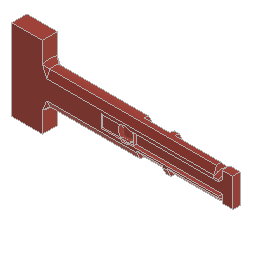
Protec2 (Autodesk Fusion 360 design; units mm, degrees)
Autodesk Fusion 360 part; units mm, degrees
sketch "profile" plane through (0, 0, 0) normal (1, 0, 0) x (0, 1, 0)
  line L0 (0, 0) -> (3.3, 0) construction
  line L1 (3.3, 0) -> (3.3, 3.3) construction
  line L2 (3.3, 3.3) -> (4.05, 3.3) construction
  line L3 (3.3, 3.3) -> (2.55, 3.3) construction
  line L4 (4.05, 3.3) -> (4.05, 4.5)
  line L5 (2.55, 3.3) -> (2.55, 2.1)
  line L6 (4.05, 3.3) -> (4.05, 2.1)
  line L7 (2.55, 3.3) -> (2.55, 4.5)
  line L8 (4.05, 4.5) -> (4.775, 4.5)
  line L9 (2.55, 2.1) -> (1.825, 2.1)
  line L10 (4.05, 2.1) -> (4.775, 2.1)
  line L11 (2.55, 4.5) -> (1.825, 4.5)
  line L12 (4.775, 4.5) -> (4.775, 5.165)
  line L13 (1.825, 2.1) -> (1.825, 1.435)
  line L14 (1.825, 4.5) -> (1.825, 5.165)
  line L15 (4.775, 2.1) -> (4.775, 1.435)
  line L16 (4.775, 5.165) -> (4.1589, 6.4863)
  line L17 (4.775, 5.165) -> (3.3, 5.165) construction
  line L18 (1.825, 1.435) -> (2.4411, 0.1137)
  line L19 (1.825, 5.165) -> (2.4411, 6.4863)
  line L20 (1.825, 5.165) -> (3.3, 5.165) construction
  line L21 (4.775, 1.435) -> (4.1589, 0.1137)
  arc A0 (4.1589, 6.4863) -> (2.4411, 6.4863) centre (3.3, 3.3) ccw
  arc A1 (2.4411, 0.1137) -> (4.1589, 0.1137) centre (3.3, 3.3) ccw
  dimension "d64" = 3.3
  dimension "d65" = 3.3
  dimension "d66" = 0.75
  dimension "d67" = 0.75
  dimension "d68" = 1.2
  dimension "d69" = 1.2
  dimension "d70" = 1.2
  dimension "d71" = 1.2
  dimension "d72" = 0.725
  dimension "d73" = 0.725
  dimension "d74" = 0.725
  dimension "d75" = 0.725
  dimension "d76" = 65
  dimension "d77" = 65
  dimension "d78" = 4.25
  dimension "d79" = 4.25
  dimension "d80" = 3.3
  constraint coincident L0.start origin
  constraint horizontal L0
  constraint perpendicular L0 L1
  constraint perpendicular L1 L2
  constraint perpendicular L1 L3
  constraint perpendicular L2 L4
  constraint perpendicular L3 L5
  constraint perpendicular L2 L6
  constraint perpendicular L3 L7
  constraint perpendicular L4 L8
  constraint perpendicular L5 L9
  constraint perpendicular L6 L10
  constraint perpendicular L7 L11
  constraint perpendicular L8 L12
  constraint perpendicular L9 L13
  constraint equal L12 L13
  constraint perpendicular L11 L14
  constraint perpendicular L10 L15
  constraint equal L14 L15
  constraint horizontal L17
  constraint equal L16 L18
  constraint parallel L16 L18
  constraint vertical L1.end L17.end
  constraint horizontal L20
  constraint equal L19 L21
  constraint parallel L19 L21
  constraint coincident L1.end L2.start
  constraint coincident L16.end A0.start
  measures "d64" distance of L0.start L0.end
  measures "d65" distance of L0.end L1.end
  measures "d66" distance of L1.end L2.end
  measures "d67" distance of L1.end L3.end
  measures "d68" distance of L2.end L4.end
  measures "d69" distance of L3.end L5.end
  measures "d70" distance of L2.end L6.end
  measures "d71" distance of L3.end L7.end
  measures "d72" distance of L4.end L8.end
  measures "d73" distance of L5.end L9.end
  measures "d74" distance of L6.end L10.end
  measures "d75" distance of L7.end L11.end
  measures "d76" angle of L16 L17
  measures "d77" angle of L19 L20
  measures "d78" distance of L16 L18
  measures "d79" distance of L19 L21
  measures "d80" radius of A0
extrude "Extrude1" add sketch "profile" against normal blind 42.57 makes body 1
ref_plane "WorkPlane1" through (-21.285, 3.3, 3.3) normal (0, -1, 0) x (0, 0, 1)
sketch "bearing hole" plane through (0, 3.3, 0) normal (0, -1, 0) x (-1, 0, 0)
  line L0 (0, 0) -> (0, -3.3) construction
  line L1 (0, -3.3) -> (20.5, -3.3) construction
  circle A0 centre (20.5, -3.3) radius 1.5
  dimension "d83" = 3.3
  dimension "d84" = 20.5
  dimension "d85" = 3
  constraint coincident L0.start origin
  constraint vertical L0
  constraint perpendicular L0 L1
  constraint coincident L1.end A0.centre
  measures "d83" distance of L0.start L0.end
  measures "d84" distance of L0.end L1.end
  measures "d85" diameter of A0
ref_plane "WorkPlane2" through (-42.57, 0, 0) normal (1, 0, 0) x (0, 1, 0)
sketch "bow" plane through (-42.57, 0, 0) normal (1, 0, 0) x (0, 1, 0)
  circle A0 centre (3.3, 3.3) radius 3.3 construction
  line L0 (4.775, 5.165) -> (4.775, 6.252)
  line L1 (4.775, 1.435) -> (4.775, 0.348)
  line L2 (1.825, 1.435) -> (1.825, 0.348)
  line L3 (1.825, 5.165) -> (1.825, 6.252)
  line L4 (4.775, 5.165) -> (4.775, 1.435)
  line L5 (1.825, 5.165) -> (1.825, 1.435)
  line L6 (4.775, 6.252) -> (4.775, 11.252)
  line L7 (1.825, 0.348) -> (1.825, -4.652)
  line L8 (4.775, 11.252) -> (1.825, 11.252)
  line L9 (1.825, 11.252) -> (1.825, 6.252)
  line L10 (1.825, -4.652) -> (4.775, -4.652)
  line L11 (4.775, -4.652) -> (4.775, 0.348)
  line L12 (2.55, 2.1) -> (2.55, 4.5) construction
  line L13 (2.55, 4.5) -> (1.825, 4.5) construction
  line L14 (1.825, 4.5) -> (1.825, 5.165) construction
  line L15 (1.825, 5.165) -> (2.4411, 6.4863) construction
  arc A1 (4.1589, 6.4863) -> (2.4411, 6.4863) centre (3.3, 3.3) ccw construction
  line L16 (4.1589, 6.4863) -> (4.775, 5.165) construction
  line L17 (4.775, 5.165) -> (4.775, 4.5) construction
  line L18 (4.775, 4.5) -> (4.05, 4.5) construction
  line L19 (4.05, 4.5) -> (4.05, 2.1) construction
  line L20 (4.05, 2.1) -> (4.775, 2.1) construction
  line L21 (4.775, 2.1) -> (4.775, 1.435) construction
  line L22 (4.775, 1.435) -> (4.1589, 0.1137) construction
  arc A2 (2.4411, 0.1137) -> (4.1589, 0.1137) centre (3.3, 3.3) ccw construction
  line L23 (2.4411, 0.1137) -> (1.825, 1.435) construction
  line L24 (1.825, 1.435) -> (1.825, 2.1) construction
  line L25 (1.825, 2.1) -> (2.55, 2.1) construction
  dimension "d86" = 5
  dimension "d87" = 5
  constraint coincident A0 L0.end
  constraint coincident A0 L1.end
  constraint coincident A0 L2.end
  constraint coincident A0 L3.end
  constraint parallel L0 L6
  constraint parallel L2 L7
  constraint perpendicular L3 L8
  constraint perpendicular L8 L9
  constraint perpendicular L1 L10
  constraint perpendicular L10 L11
  constraint coincident L0.start L4.start
  constraint coincident A0 A1.start
  constraint coincident A0 L15.end
  constraint coincident A0 A2.start
  constraint vertical L9
  constraint vertical L6
  constraint vertical L11
  constraint vertical L7
  constraint vertical L4
  constraint vertical L5
  constraint coincident L2.start L5.end
  constraint coincident L3.start L5.start
  constraint coincident L1.start L4.end
  measures "d86" distance of L0.end L6.end
  measures "d87" distance of L2.end L7.end
sketch "bearing hole and shaft strength" plane through (-42.57, 0, 0) normal (1, 0, 0) x (0, 1, 0)
  line L0 (2.55, 2.1) -> (2.55, 4.5)
  line L1 (4.05, 4.5) -> (4.05, 2.1)
  line L2 (2.55, 4.5) -> (1.825, 4.5)
  line L3 (1.825, 2.1) -> (2.55, 2.1)
  line L4 (4.05, 2.1) -> (4.775, 2.1)
  line L5 (4.775, 4.5) -> (4.05, 4.5)
  line L6 (2.125, 4.5) -> (2.125, 2.1)
  line L7 (4.475, 4.5) -> (4.475, 2.1)
  line L8 (1.825, 4.5) -> (1.825, 2.1)
  line L9 (4.775, 2.1) -> (4.775, 4.5)
  dimension "d89" = 0.425
  dimension "d90" = 0.425
  constraint coincident L2 L6.start
  constraint coincident L3 L6.end
  constraint perpendicular L3 L6
  constraint coincident L5 L7.start
  constraint coincident L4 L7.end
  constraint perpendicular L4 L7
  constraint coincident L2.end L8.start
  constraint coincident L3.start L8.end
  constraint coincident L4.end L9.start
  constraint coincident L5.start L9.end
  measures "d89" distance of L0 L6
  measures "d90" distance of L1 L7
extrude "Extrude2" add sketch "bow" along normal blind 6 bodies 1
extrude "Extrude3" add sketch "bearing hole and shaft strength" along normal blind 23.625 contours L0 L2 L3 L6 | L1 L4 L5 L7 bodies 1
extrude "Extrude4" add sketch "bearing hole and shaft strength" along normal blind 17.5 contours L2 L3 L6 L8 | L4 L5 L7 L9 bodies 1
chamfer "Chamfer1" distance 0.85 angle 45 6 edges at (-36.57, 2.1331, 5.8256) (-36.57, 3.3, 6.6) (-36.57, 2.1331, 0.7744) (-36.57, 4.4669, 5.8256) (-36.57, 4.4669, 0.7744) (-36.57, 3.3, 0) on bodies 1
extrude "Extrude5" cut sketch "bearing hole" along normal through all and the other way through all bodies 1
sketch "bearing" plane through (0, 3.3, 0) normal (0, -1, 0) x (-1, 0, 0)
  circle A0 centre (20.5, -3.3) radius 1.25
  point P0 (20.5, -3.3)
  dimension "d99" = 2.5
  constraint coincident P0 A0.centre
  measures "d99" diameter of A0
ref_plane "WorkPlane3" through (-20.5, 4.775, 3.3) normal (-1, 0, 0) x (0, -1, 0)
sketch "bearing post" plane through (-20.5, 0, 0) normal (-1, 0, 0) x (0, -1, 0)
  circle A0 centre (-3.3, 3.3) radius 0.3
  point P0 (-3.3, 3.3)
  dimension "d105" = 0.6
  constraint coincident P0 A0.centre
  measures "d105" diameter of A0
extrude "Extrude6" add sketch "bearing" along normal mid plane 2.5 separate body makes body 2
fillet "Fillet1" radius 1.25 2 edges at (-19.3346, 2.05, 3.752) (-19.3346, 4.55, 2.848) on bodies 2
extrude "Extrude7" add sketch "bearing post" along normal up to surface end surface at (-21.2817, 3.6917, 4.5802) on bodies 1 bodies 1 2
sketch "bearing retention" plane through (0, 2.125, 0) normal (0, -1, 0) x (1, 0, 0)
  arc A0 (-21.4, 4.5) -> (-21.4, 2.1) centre (-20.5, 3.3) ccw
  line L0 (-21.4, 4.5) -> (-25.07, 4.5)
  line L1 (-25.07, 4.5) -> (-25.07, 2.1)
  line L2 (-25.07, 2.1) -> (-21.4, 2.1)
  arc A1 (-21.4, 2.1) -> (-19.6, 2.1) centre (-20.5, 3.3) ccw
  arc A2 (-19.6, 4.5) -> (-21.4, 4.5) centre (-20.5, 3.3) ccw
  line L3 (-21.3292, 2.05) -> (-19.6708, 2.05) construction
  line L4 (-21.3292, 2.05) -> (-21.3292, 2.225)
  line L5 (-21.3292, 2.225) -> (-19.6708, 2.225)
  line L6 (-19.6708, 2.225) -> (-19.6708, 2.05)
  line L7 (-21.3292, 4.55) -> (-19.6708, 4.55) construction
  line L8 (-21.3292, 4.55) -> (-21.3292, 4.375)
  line L9 (-21.3292, 4.375) -> (-19.6708, 4.375)
  line L10 (-19.6708, 4.375) -> (-19.6708, 4.55)
  point P0 (-20.5, 1.8)
  point P1 (-20.5, 4.8)
  dimension "d108" = 0.25
  dimension "d109" = 0.175
  dimension "d110" = 0.175
  constraint midpoint A2 P1
  constraint coincident A1 L3.start
  constraint coincident A1 L3.end
  constraint horizontal L3
  constraint perpendicular L3 L4
  constraint perpendicular L4 L5
  constraint perpendicular L3 L6
  constraint coincident A2 L7.start
  constraint coincident A2 L7.end
  constraint horizontal L7
  constraint equal L3 L7
  constraint perpendicular L7 L8
  constraint perpendicular L8 L9
  constraint perpendicular L7 L10
  constraint midpoint A1 P0
  measures "d108" distance of P0 L3
  measures "d109" distance of L3.start L4.end
  measures "d110" distance of L7.start L8.end
extrude "Extrude8" add sketch "bearing retention" against normal blind 0.35 contours A1 L4 L5 L6 | A2 L8 L9 L10 bodies 1
fillet "Fillet2" radius 0.175 2 faces at (-20.7764, 2.2417, 2.225) (-20.7764, 2.2417, 4.375) on bodies 1
mirror "Mirror1" about plane through (-21.285, 3.3, 3.3) normal (0, -1, 0) of "Extrude8", "Fillet2"
sketch "tip" plane through (0, 0, 0) normal (1, 0, 0) x (0, 1, 0)
  line L0 (0, 0) -> (3.3, 0) construction
  line L1 (3.3, 0) -> (3.3, 3.3) construction
  line L2 (3.3, 3.3) -> (4.05, 3.3) construction
  line L3 (3.3, 3.3) -> (2.55, 3.3) construction
  line L4 (4.05, 3.3) -> (4.05, 6.1013)
  line L5 (2.55, 3.3) -> (2.55, 0.4987)
  line L6 (4.05, 3.3) -> (4.05, 0.4987)
  line L7 (2.55, 3.3) -> (2.55, 6.1013)
  arc A0 (4.05, 6.1013) -> (2.55, 6.1013) centre (3.3, 3.3) ccw
  arc A1 (2.55, 0.4987) -> (4.05, 0.4987) centre (3.3, 3.3) ccw
  circle A2 centre (3.3, 3.3) radius 3.3
  dimension "d117" = 3.3
  dimension "d118" = 3.3
  dimension "d119" = 0.75
  dimension "d120" = 0.75
  dimension "d121" = 2.9
  dimension "d122" = 6.6
  constraint coincident L0.start origin
  constraint horizontal L0
  constraint perpendicular L0 L1
  constraint perpendicular L1 L2
  constraint perpendicular L1 L3
  constraint perpendicular L2 L4
  constraint perpendicular L3 L5
  constraint perpendicular L2 L6
  constraint perpendicular L3 L7
  constraint equal L5 L7
  constraint equal L6 L7
  constraint equal L4 L6
  constraint coincident L1.end L2.start
  constraint concentric A0 A2
  measures "d117" distance of L0.start L0.end
  measures "d118" distance of L0.end L1.end
  measures "d119" distance of L1.end L2.end
  measures "d120" distance of L1.end L3.end
  measures "d121" radius of A0
  measures "d122" diameter of A2
sketch "profiled 0 cut" plane through (0, 0, 0) normal (1, 0, 0) x (0, 1, 0)
  line L0 (2.55, 4.5) -> (1.825, 4.5)
  line L1 (2.55, 3.3) -> (2.55, 4.5)
  line L2 (2.55, 3.3) -> (2.55, 2.1)
  line L3 (2.55, 2.1) -> (1.825, 2.1)
  line L4 (4.05, 3.3) -> (4.05, 4.5)
  line L5 (4.05, 4.5) -> (4.775, 4.5)
  line L6 (4.05, 3.3) -> (4.05, 2.1)
  line L7 (4.05, 2.1) -> (4.775, 2.1)
  line L8 (4.775, 4.5) -> (4.775, 4.8293)
  line L9 (1.825, 2.1) -> (1.825, 1.7707)
  line L10 (4.775, 2.1) -> (4.775, 1.7707)
  line L11 (1.825, 4.5) -> (1.825, 4.8293)
  line L12 (4.775, 4.8293) -> (4.7747, 4.83)
  line L13 (4.775, 4.8293) -> (3.3, 4.8293) construction
  line L14 (1.825, 1.7707) -> (1.8253, 1.77)
  line L15 (1.825, 4.8293) -> (1.8253, 4.83)
  line L16 (1.825, 4.8293) -> (3.3, 4.8293) construction
  line L17 (4.775, 1.7707) -> (4.7747, 1.77)
  arc A0 (4.7747, 4.83) -> (1.8253, 4.83) centre (3.3, 3.3) ccw
  arc A1 (1.8253, 1.77) -> (4.7747, 1.77) centre (3.3, 3.3) ccw
  circle A2 centre (3.3, 3.3) radius 4.125
  point P0 (3.3, 3.3)
  dimension "d153" = 65
  dimension "d154" = 65
  dimension "d155" = 3.9663
  dimension "d156" = 3.9663
  dimension "d157" = 2.125
  dimension "d158" = 8.25
  constraint coincident L5.end L8.start
  constraint perpendicular L5 L8
  constraint coincident L3.end L9.start
  constraint perpendicular L3 L9
  constraint equal L8 L9
  constraint coincident L7.end L10.start
  constraint perpendicular L7 L10
  constraint coincident L0.end L11.start
  constraint perpendicular L0 L11
  constraint equal L10 L11
  constraint horizontal L13
  constraint vertical P0 L13.end
  constraint equal L12 L14
  constraint parallel L12 L14
  constraint horizontal L16
  constraint equal L15 L17
  constraint parallel L15 L17
  constraint coincident P0 A0.centre
  constraint coincident L12.end A0.start
  measures "d153" angle of L12 L13
  measures "d154" angle of L15 L16
  measures "d155" distance of L12 L14
  measures "d156" distance of L15 L17
  measures "d157" radius of A0
  measures "d158" diameter of A2
sketch "Sketch9" plane through (0, 0, 0) normal (1, 0, 0) x (0, 1, 0)
  line L0 (4.05, 4.5) -> (4.775, 4.5)
  line L1 (4.05, 3.3) -> (4.05, 4.5)
  line L2 (4.05, 3.3) -> (4.05, 2.1)
  line L3 (4.05, 2.1) -> (4.775, 2.1)
  line L4 (2.55, 2.1) -> (1.825, 2.1)
  line L5 (2.55, 3.3) -> (2.55, 2.1)
  line L6 (2.55, 3.3) -> (2.55, 4.5)
  line L7 (2.55, 4.5) -> (1.825, 4.5)
  line L8 (4.775, 4.5) -> (4.775, 4.8481)
  line L9 (1.825, 2.1) -> (1.825, 1.7519)
  line L10 (4.775, 4.8481) -> (3.305, 6.6)
  line L11 (4.775, 4.8481) -> (3.3, 4.8481) construction
  line L12 (1.825, 1.7519) -> (3.295, 0)
  line L13 (1.825, 4.5) -> (1.825, 5.165)
  line L14 (4.775, 2.1) -> (4.775, 1.435)
  line L15 (1.825, 5.165) -> (2.4411, 6.4863)
  line L16 (1.825, 5.165) -> (3.3, 5.165) construction
  line L17 (4.775, 1.435) -> (4.1589, 0.1137)
  arc A0 (3.305, 6.6) -> (2.4411, 6.4863) centre (3.3, 3.3) ccw
  arc A1 (3.295, 0) -> (4.1589, 0.1137) centre (3.3, 3.3) ccw
  circle A2 centre (3.3, 3.3) radius 4.125
  point P0 (3.3, 3.3)
  dimension "d123" = 50
  dimension "d124" = 65
  dimension "d125" = 3.3
  dimension "d126" = 4.25
  dimension "d127" = 4.25
  dimension "d128" = 8.25
  constraint coincident L0.end L8.start
  constraint perpendicular L0 L8
  constraint coincident L4.end L9.start
  constraint perpendicular L4 L9
  constraint equal L8 L9
  constraint horizontal L11
  constraint vertical P0 L11.end
  constraint parallel L10 L12
  constraint coincident L7.end L13.start
  constraint perpendicular L7 L13
  constraint coincident L3.end L14.start
  constraint perpendicular L3 L14
  constraint equal L13 L14
  constraint horizontal L16
  constraint parallel L15 L17
  constraint equal L15 L17
  constraint equal L10 L12
  constraint coincident P0 A0.centre
  constraint coincident L10.end A0.start
  constraint equal A0 A1
  constraint vertical L16.end P0
  constraint concentric A0 A2
  measures "d123" angle of L10 L11
  measures "d124" angle of L15 L16
  measures "d125" radius of A0
  measures "d126" distance of L10 L12
  measures "d127" distance of L15 L17
  measures "d128" diameter of A2
sketch "Sketch10" plane through (0, 0, 0) normal (1, 0, 0) x (0, 1, 0)
  line L0 (2.55, 4.5) -> (1.825, 4.5)
  line L1 (2.55, 3.3) -> (2.55, 4.5)
  line L2 (4.05, 4.5) -> (4.775, 4.5)
  line L3 (4.05, 3.3) -> (4.05, 4.5)
  line L4 (4.05, 2.1) -> (4.775, 2.1)
  line L5 (4.05, 3.3) -> (4.05, 2.1)
  line L6 (2.55, 3.3) -> (2.55, 2.1)
  line L7 (2.55, 2.1) -> (1.825, 2.1)
  line L8 (4.775, 4.5) -> (4.775, 4.8481)
  line L9 (1.825, 2.1) -> (1.825, 1.7519)
  line L10 (1.825, 4.5) -> (1.825, 5.165)
  line L11 (4.775, 2.1) -> (4.775, 1.435)
  line L12 (4.775, 4.8481) -> (3.305, 6.6)
  line L13 (4.775, 4.8481) -> (3.3, 4.8481) construction
  line L14 (1.825, 1.7519) -> (3.295, 0)
  line L15 (1.825, 5.165) -> (2.4411, 6.4863)
  line L16 (1.825, 5.165) -> (3.3, 5.165) construction
  line L17 (4.775, 1.435) -> (4.1589, 0.1137)
  arc A0 (3.305, 6.6) -> (2.4411, 6.4863) centre (3.3, 3.3) ccw
  arc A1 (3.295, 0) -> (4.1589, 0.1137) centre (3.3, 3.3) ccw
  circle A2 centre (3.3, 3.3) radius 4.125
  point P0 (3.3, 3.3)
  dimension "d129" = 50
  dimension "d130" = 65
  dimension "d131" = 4.25
  dimension "d132" = 4.25
  dimension "d133" = 3.3
  dimension "d134" = 8.25
  constraint coincident L2.end L8.start
  constraint perpendicular L2 L8
  constraint coincident L7.end L9.start
  constraint perpendicular L7 L9
  constraint equal L8 L9
  constraint coincident L0.end L10.start
  constraint perpendicular L0 L10
  constraint coincident L4.end L11.start
  constraint perpendicular L4 L11
  constraint equal L10 L11
  constraint horizontal L13
  constraint equal L12 L14
  constraint parallel L12 L14
  constraint vertical P0 L13.end
  constraint horizontal L16
  constraint vertical P0 L16.end
  constraint equal L15 L17
  constraint parallel L15 L17
  constraint coincident P0 A0.centre
  constraint coincident L12.end A0.start
  constraint equal A0 A1
  constraint concentric A1 A2
  measures "d129" angle of L12 L13
  measures "d130" angle of L15 L16
  measures "d131" distance of L12 L14
  measures "d132" distance of L15 L17
  measures "d133" radius of A0
  measures "d134" diameter of A2
sketch "Sketch11" plane through (0, 0, 0) normal (1, 0, 0) x (0, 1, 0)
  line L0 (4.05, 4.5) -> (4.775, 4.5)
  line L1 (4.05, 3.3) -> (4.05, 4.5)
  line L2 (4.05, 3.3) -> (4.05, 2.1)
  line L3 (4.05, 2.1) -> (4.775, 2.1)
  line L4 (2.55, 3.3) -> (2.55, 4.5)
  line L5 (2.55, 3.3) -> (2.55, 2.1)
  line L6 (2.55, 2.1) -> (1.825, 2.1)
  line L7 (2.55, 4.5) -> (1.825, 4.5)
  line L8 (4.775, 4.5) -> (4.775, 4.8481)
  line L9 (1.825, 2.1) -> (1.825, 1.7519)
  line L10 (1.825, 4.5) -> (1.825, 5.165)
  line L11 (4.775, 2.1) -> (4.775, 1.435)
  line L12 (4.775, 4.8481) -> (3.305, 6.6)
  line L13 (4.775, 4.8481) -> (3.3, 4.8481) construction
  line L14 (1.825, 1.7519) -> (3.295, 0)
  line L15 (1.825, 5.165) -> (2.4411, 6.4863)
  line L16 (1.825, 5.165) -> (3.3, 5.165) construction
  line L17 (4.775, 1.435) -> (4.1589, 0.1137)
  arc A0 (3.305, 6.6) -> (2.4411, 6.4863) centre (3.3, 3.3) ccw
  arc A1 (3.295, 0) -> (4.1589, 0.1137) centre (3.3, 3.3) ccw
  circle A2 centre (3.3, 3.3) radius 4.125
  point P0 (3.3, 3.3)
  dimension "d135" = 50
  dimension "d136" = 65
  dimension "d137" = 4.25
  dimension "d138" = 4.25
  dimension "d139" = 3.3
  dimension "d140" = 8.25
  constraint coincident L0.end L8.start
  constraint perpendicular L0 L8
  constraint coincident L6.end L9.start
  constraint perpendicular L6 L9
  constraint equal L8 L9
  constraint coincident L7.end L10.start
  constraint perpendicular L7 L10
  constraint coincident L3.end L11.start
  constraint perpendicular L3 L11
  constraint equal L10 L11
  constraint horizontal L13
  constraint parallel L12 L14
  constraint equal L12 L14
  constraint vertical P0 L13.end
  constraint horizontal L16
  constraint vertical P0 L16.end
  constraint equal L15 L17
  constraint parallel L15 L17
  constraint coincident P0 A0.centre
  constraint coincident L12.end A0.start
  constraint equal A0 A1
  constraint concentric A1 A2
  measures "d135" angle of L12 L13
  measures "d136" angle of L15 L16
  measures "d137" distance of L12 L14
  measures "d138" distance of L15 L17
  measures "d139" radius of A0
  measures "d140" diameter of A2
sketch "Sketch12" plane through (0, 0, 0) normal (1, 0, 0) x (0, 1, 0)
  line L0 (2.55, 4.5) -> (1.825, 4.5)
  line L1 (2.55, 3.3) -> (2.55, 4.5)
  line L2 (2.55, 3.3) -> (2.55, 2.1)
  line L3 (2.55, 2.1) -> (1.825, 2.1)
  line L4 (4.05, 3.3) -> (4.05, 4.5)
  line L5 (4.05, 4.5) -> (4.775, 4.5)
  line L6 (4.05, 3.3) -> (4.05, 2.1)
  line L7 (4.05, 2.1) -> (4.775, 2.1)
  line L8 (4.775, 4.5) -> (4.775, 4.8481)
  line L9 (1.825, 2.1) -> (1.825, 1.7519)
  line L10 (1.825, 4.5) -> (1.825, 5.165)
  line L11 (4.775, 2.1) -> (4.775, 1.435)
  line L12 (4.775, 4.8481) -> (3.305, 6.6)
  line L13 (4.775, 4.8481) -> (3.3, 4.8481) construction
  line L14 (1.825, 1.7519) -> (3.295, 0)
  line L15 (1.825, 5.165) -> (2.4411, 6.4863)
  line L16 (1.825, 5.165) -> (3.3, 5.165) construction
  line L17 (4.775, 1.435) -> (4.1589, 0.1137)
  arc A0 (3.305, 6.6) -> (2.4411, 6.4863) centre (3.3, 3.3) ccw
  arc A1 (3.295, 0) -> (4.1589, 0.1137) centre (3.3, 3.3) ccw
  circle A2 centre (3.3, 3.3) radius 4.125
  point P0 (3.3, 3.3)
  dimension "d141" = 50
  dimension "d142" = 65
  dimension "d143" = 4.25
  dimension "d144" = 4.25
  dimension "d145" = 3.3
  dimension "d146" = 8.25
  constraint coincident L5.end L8.start
  constraint perpendicular L5 L8
  constraint coincident L3.end L9.start
  constraint perpendicular L3 L9
  constraint equal L8 L9
  constraint coincident L0.end L10.start
  constraint perpendicular L0 L10
  constraint coincident L7.end L11.start
  constraint perpendicular L7 L11
  constraint equal L10 L11
  constraint horizontal L13
  constraint vertical P0 L13.end
  constraint equal L12 L14
  constraint parallel L12 L14
  constraint horizontal L16
  constraint vertical P0 L16.end
  constraint parallel L15 L17
  constraint equal L15 L17
  constraint coincident P0 A0.centre
  constraint coincident L12.end A0.start
  constraint equal A0 A1
  measures "d141" angle of L12 L13
  measures "d142" angle of L15 L16
  measures "d143" distance of L12 L14
  measures "d144" distance of L15 L17
  measures "d145" radius of A0
  measures "d146" diameter of A2
sketch "Sketch13" plane through (0, 0, 0) normal (1, 0, 0) x (0, 1, 0)
  line L0 (2.55, 4.5) -> (1.825, 4.5)
  line L1 (2.55, 3.3) -> (2.55, 4.5)
  line L2 (2.55, 3.3) -> (2.55, 2.1)
  line L3 (2.55, 2.1) -> (1.825, 2.1)
  line L4 (4.05, 2.1) -> (4.775, 2.1)
  line L5 (4.05, 3.3) -> (4.05, 2.1)
  line L6 (4.05, 3.3) -> (4.05, 4.5)
  line L7 (4.05, 4.5) -> (4.775, 4.5)
  line L8 (4.775, 4.5) -> (4.775, 4.8481)
  line L9 (1.825, 2.1) -> (1.825, 1.7519)
  line L10 (1.825, 4.5) -> (1.825, 5.165)
  line L11 (4.775, 2.1) -> (4.775, 1.435)
  line L12 (4.775, 4.8481) -> (3.305, 6.6)
  line L13 (4.775, 4.8481) -> (3.3, 4.8481) construction
  line L14 (1.825, 1.7519) -> (3.295, 0)
  line L15 (1.825, 5.165) -> (2.4411, 6.4863)
  line L16 (1.825, 5.165) -> (3.3, 5.165) construction
  line L17 (4.775, 1.435) -> (4.1589, 0.1137)
  arc A0 (3.305, 6.6) -> (2.4411, 6.4863) centre (3.3, 3.3) ccw
  arc A1 (3.295, 0) -> (4.1589, 0.1137) centre (3.3, 3.3) ccw
  circle A2 centre (3.3, 3.3) radius 4.125
  point P0 (3.3, 3.3)
  dimension "d147" = 50
  dimension "d148" = 65
  dimension "d149" = 4.25
  dimension "d150" = 4.25
  dimension "d151" = 3.3
  dimension "d152" = 8.25
  constraint coincident L7.end L8.start
  constraint perpendicular L7 L8
  constraint coincident L3.end L9.start
  constraint perpendicular L3 L9
  constraint equal L8 L9
  constraint coincident L0.end L10.start
  constraint perpendicular L0 L10
  constraint coincident L4.end L11.start
  constraint perpendicular L4 L11
  constraint equal L10 L11
  constraint horizontal L13
  constraint vertical P0 L13.end
  constraint equal L12 L14
  constraint parallel L12 L14
  constraint horizontal L16
  constraint vertical P0 L16.end
  constraint parallel L15 L17
  constraint equal L15 L17
  constraint coincident P0 A0.centre
  constraint coincident L12.end A0.start
  constraint equal A0 A1
  constraint concentric A1 A2
  measures "d147" angle of L12 L13
  measures "d148" angle of L15 L16
  measures "d149" distance of L12 L14
  measures "d150" distance of L15 L17
  measures "d151" radius of A0
  measures "d152" diameter of A2
sketch "Sketch15" plane through (0, 0, 0) normal (1, 0, 0) x (0, 1, 0)
  line L0 (2.55, 4.5) -> (1.825, 4.5)
  line L1 (2.55, 3.3) -> (2.55, 4.5)
  line L2 (2.55, 3.3) -> (2.55, 2.1)
  line L3 (2.55, 2.1) -> (1.825, 2.1)
  line L4 (4.05, 3.3) -> (4.05, 4.5)
  line L5 (4.05, 4.5) -> (4.775, 4.5)
  line L6 (4.05, 3.3) -> (4.05, 2.1)
  line L7 (4.05, 2.1) -> (4.775, 2.1)
  line L8 (4.775, 4.5) -> (4.775, 4.8481)
  line L9 (1.825, 2.1) -> (1.825, 1.7519)
  line L10 (1.825, 4.5) -> (1.825, 5.165)
  line L11 (4.775, 2.1) -> (4.775, 1.435)
  line L12 (4.775, 4.8481) -> (3.305, 6.6)
  line L13 (4.775, 4.8481) -> (3.3, 4.8481) construction
  line L14 (1.825, 1.7519) -> (3.295, 0)
  line L15 (1.825, 5.165) -> (2.4411, 6.4863)
  line L16 (1.825, 5.165) -> (3.3, 5.165) construction
  line L17 (4.775, 1.435) -> (4.1589, 0.1137)
  arc A0 (3.305, 6.6) -> (2.4411, 6.4863) centre (3.3, 3.3) ccw
  arc A1 (3.295, 0) -> (4.1589, 0.1137) centre (3.3, 3.3) ccw
  circle A2 centre (3.3, 3.3) radius 4.125
  point P0 (3.3, 3.3)
  dimension "d159" = 50
  dimension "d160" = 65
  dimension "d161" = 4.25
  dimension "d162" = 4.25
  dimension "d163" = 3.3
  dimension "d164" = 8.25
  constraint coincident L5.end L8.start
  constraint perpendicular L5 L8
  constraint coincident L3.end L9.start
  constraint perpendicular L3 L9
  constraint equal L8 L9
  constraint coincident L0.end L10.start
  constraint perpendicular L0 L10
  constraint coincident L7.end L11.start
  constraint perpendicular L7 L11
  constraint equal L10 L11
  constraint horizontal L13
  constraint vertical P0 L13.end
  constraint equal L12 L14
  constraint parallel L12 L14
  constraint horizontal L16
  constraint vertical P0 L16.end
  constraint equal L15 L17
  constraint parallel L15 L17
  constraint coincident P0 A0.centre
  constraint coincident L12.end A0.start
  constraint equal A0 A1
  constraint concentric A1 A2
  measures "d159" angle of L12 L13
  measures "d160" angle of L15 L16
  measures "d161" distance of L12 L14
  measures "d162" distance of L15 L17
  measures "d163" radius of A0
  measures "d164" diameter of A2
sketch "Sketch16" plane through (0, 0, 0) normal (1, 0, 0) x (0, 1, 0)
  line L0 (2.55, 4.5) -> (1.825, 4.5)
  line L1 (2.55, 3.3) -> (2.55, 4.5)
  line L2 (2.55, 3.3) -> (2.55, 2.1)
  line L3 (2.55, 2.1) -> (1.825, 2.1)
  line L4 (4.05, 3.3) -> (4.05, 2.1)
  line L5 (4.05, 2.1) -> (4.775, 2.1)
  line L6 (4.05, 4.5) -> (4.775, 4.5)
  line L7 (4.05, 3.3) -> (4.05, 4.5)
  line L8 (4.775, 4.5) -> (4.775, 4.8481)
  line L9 (1.825, 2.1) -> (1.825, 1.7519)
  line L10 (1.825, 4.5) -> (1.825, 5.165)
  line L11 (4.775, 2.1) -> (4.775, 1.435)
  line L12 (4.775, 4.8481) -> (3.305, 6.6)
  line L13 (4.775, 4.8481) -> (3.3, 4.8481) construction
  line L14 (1.825, 1.7519) -> (3.295, 0)
  line L15 (1.825, 5.165) -> (2.4411, 6.4863)
  line L16 (1.825, 5.165) -> (3.3, 5.165) construction
  line L17 (4.775, 1.435) -> (4.1589, 0.1137)
  arc A0 (3.305, 6.6) -> (2.4411, 6.4863) centre (3.3, 3.3) ccw
  arc A1 (3.295, 0) -> (4.1589, 0.1137) centre (3.3, 3.3) ccw
  circle A2 centre (3.3, 3.3) radius 4.125
  point P0 (3.3, 3.3)
  dimension "d165" = 50
  dimension "d166" = 65
  dimension "d167" = 4.25
  dimension "d168" = 4.25
  dimension "d169" = 3.3
  dimension "d170" = 8.25
  constraint coincident L6.end L8.start
  constraint perpendicular L6 L8
  constraint coincident L3.end L9.start
  constraint perpendicular L3 L9
  constraint equal L8 L9
  constraint coincident L0.end L10.start
  constraint perpendicular L0 L10
  constraint coincident L5.end L11.start
  constraint perpendicular L5 L11
  constraint equal L10 L11
  constraint horizontal L13
  constraint vertical P0 L13.end
  constraint equal L12 L14
  constraint parallel L12 L14
  constraint horizontal L16
  constraint vertical P0 L16.end
  constraint equal L15 L17
  constraint parallel L15 L17
  constraint coincident P0 A0.centre
  constraint coincident L12.end A0.start
  constraint equal A0 A1
  measures "d165" angle of L12 L13
  measures "d166" angle of L15 L16
  measures "d167" distance of L12 L14
  measures "d168" distance of L15 L17
  measures "d169" radius of A0
  measures "d170" diameter of A2
sketch "Sketch17" plane through (0, 0, 0) normal (1, 0, 0) x (0, 1, 0)
  line L0 (2.55, 4.5) -> (1.825, 4.5)
  line L1 (2.55, 3.3) -> (2.55, 4.5)
  line L2 (2.55, 3.3) -> (2.55, 2.1)
  line L3 (2.55, 2.1) -> (1.825, 2.1)
  line L4 (4.05, 3.3) -> (4.05, 4.5)
  line L5 (4.05, 3.3) -> (4.05, 2.1)
  line L6 (4.05, 2.1) -> (4.775, 2.1)
  line L7 (4.05, 4.5) -> (4.775, 4.5)
  line L8 (4.775, 4.5) -> (4.775, 4.8481)
  line L9 (1.825, 2.1) -> (1.825, 1.7519)
  line L10 (1.825, 4.5) -> (1.825, 5.165)
  line L11 (4.775, 2.1) -> (4.775, 1.435)
  line L12 (4.775, 4.8481) -> (3.305, 6.6)
  line L13 (4.775, 4.8481) -> (3.3, 4.8481) construction
  line L14 (1.825, 1.7519) -> (3.295, 0)
  line L15 (1.825, 5.165) -> (2.4411, 6.4863)
  line L16 (1.825, 5.165) -> (3.3, 5.165) construction
  line L17 (4.775, 1.435) -> (4.1589, 0.1137)
  arc A0 (3.305, 6.6) -> (2.4411, 6.4863) centre (3.3, 3.3) ccw
  arc A1 (3.295, 0) -> (4.1589, 0.1137) centre (3.3, 3.3) ccw
  circle A2 centre (3.3, 3.3) radius 4.125
  point P0 (3.3, 3.3)
  dimension "d171" = 50
  dimension "d172" = 65
  dimension "d173" = 4.25
  dimension "d174" = 4.25
  dimension "d175" = 3.3
  dimension "d176" = 8.25
  constraint coincident L7.end L8.start
  constraint perpendicular L7 L8
  constraint coincident L3.end L9.start
  constraint perpendicular L3 L9
  constraint equal L8 L9
  constraint coincident L0.end L10.start
  constraint perpendicular L0 L10
  constraint coincident L6.end L11.start
  constraint perpendicular L6 L11
  constraint equal L10 L11
  constraint horizontal L13
  constraint vertical P0 L13.end
  constraint parallel L12 L14
  constraint equal L12 L14
  constraint horizontal L16
  constraint vertical P0 L16.end
  constraint equal L15 L17
  constraint parallel L15 L17
  constraint coincident P0 A0.centre
  constraint coincident L12.end A0.start
  constraint equal A0 A1
  measures "d171" angle of L12 L13
  measures "d172" angle of L15 L16
  measures "d173" distance of L12 L14
  measures "d174" distance of L15 L17
  measures "d175" radius of A0
  measures "d176" diameter of A2
sketch "Sketch18" plane through (0, 0, 0) normal (1, 0, 0) x (0, 1, 0)
  line L0 (4.05, 4.5) -> (4.775, 4.5)
  line L1 (4.05, 3.3) -> (4.05, 4.5)
  line L2 (4.05, 3.3) -> (4.05, 2.1)
  line L3 (2.55, 3.3) -> (2.55, 2.1)
  line L4 (2.55, 3.3) -> (2.55, 4.5)
  line L5 (2.55, 4.5) -> (1.825, 4.5)
  line L6 (2.55, 2.1) -> (1.825, 2.1)
  line L7 (4.05, 2.1) -> (4.775, 2.1)
  line L8 (4.775, 4.5) -> (4.775, 4.8481)
  line L9 (1.825, 2.1) -> (1.825, 1.7519)
  line L10 (1.825, 4.5) -> (1.825, 5.165)
  line L11 (4.775, 2.1) -> (4.775, 1.435)
  line L12 (4.775, 4.8481) -> (3.305, 6.6)
  line L13 (4.775, 4.8481) -> (3.3, 4.8481) construction
  line L14 (1.825, 1.7519) -> (3.295, 0)
  line L15 (1.825, 5.165) -> (2.4411, 6.4863)
  line L16 (1.825, 5.165) -> (3.3, 5.165) construction
  line L17 (4.775, 1.435) -> (4.1589, 0.1137)
  arc A0 (3.305, 6.6) -> (2.4411, 6.4863) centre (3.3, 3.3) ccw
  arc A1 (3.295, 0) -> (4.1589, 0.1137) centre (3.3, 3.3) ccw
  circle A2 centre (3.3, 3.3) radius 4.125
  point P0 (3.3, 3.3)
  dimension "d177" = 50
  dimension "d178" = 65
  dimension "d179" = 4.25
  dimension "d180" = 4.25
  dimension "d181" = 3.3
  dimension "d182" = 8.25
  constraint coincident L0.end L8.start
  constraint perpendicular L0 L8
  constraint coincident L6.end L9.start
  constraint perpendicular L6 L9
  constraint equal L8 L9
  constraint coincident L5.end L10.start
  constraint perpendicular L5 L10
  constraint coincident L7.end L11.start
  constraint perpendicular L7 L11
  constraint equal L10 L11
  constraint horizontal L13
  constraint vertical P0 L13.end
  constraint equal L12 L14
  constraint parallel L12 L14
  constraint horizontal L16
  constraint vertical P0 L16.end
  constraint equal L15 L17
  constraint parallel L15 L17
  constraint coincident P0 A0.centre
  constraint coincident L12.end A0.start
  constraint equal A0 A1
  constraint concentric A1 A2
  measures "d177" angle of L12 L13
  measures "d178" angle of L15 L16
  measures "d179" distance of L12 L14
  measures "d180" distance of L15 L17
  measures "d181" radius of A0
  measures "d182" diameter of A2
extrude "Extrude9" cut sketch "profiled 0 cut" along normal mid plane 1 from surface at -2.57 bodies 1
extrude "Extrude10" cut sketch "tip" against normal blind 2.07 bodies 1
extrude "Extrude11" cut sketch "Sketch9" along normal mid plane 2 from surface at -3.57 bodies 1
extrude "Extrude12" cut sketch "Sketch10" along normal mid plane 2 from surface at -5.07 bodies 1
extrude "Extrude13" cut sketch "Sketch11" along normal mid plane 2 from surface at -6.57 bodies 1
extrude "Extrude14" cut sketch "Sketch12" along normal mid plane 2 from surface at -8.07 bodies 1
extrude "Extrude15" cut sketch "Sketch13" along normal mid plane 2 from surface at -9.57 bodies 1
extrude "Extrude16" cut sketch "Sketch15" along normal mid plane 2 from surface at -11.07 bodies 1
extrude "Extrude17" cut sketch "Sketch16" along normal mid plane 2 from surface at -14.07 bodies 1
extrude "Extrude18" cut sketch "Sketch17" along normal mid plane 2 from surface at -15.57 bodies 1
extrude "Extrude19" cut sketch "Sketch18" along normal mid plane 2 from surface at -17.07 bodies 1
equation "pos_1 = round($1)"
equation "cut_1 = if(pos_1 == 1; 1; if(pos_1 == 2; 2; if(pos_1 == 3; 3; if(pos_1 == 4; 4; if(pos_1 == 5; 5; 6)))))"
equation "right_angle_1 = if(cut_1 == 1; 50 deg; if(cut_1 == 2; 65 deg; if(cut_1 == 3; 35 deg; if(cut_1 == 4; 50 deg; if(cut_1 == 5; 65 deg; 65 deg)))))"
equation "left_angle_1 = if(cut_1 == 1; 65 deg; if(cut_1 == 2; 50 deg; if(cut_1 == 3; 65 deg; if(cut_1 == 4; 50 deg; if(cut_1 == 5; 35 deg; 65 deg)))))"
equation "end_diameters_1 = if(( cut_1 == 1 ) or ( cut_1 == 2 ); 3.3 mm; if(( cut_1 == 3 ) or ( cut_1 == 4 ) or ( cut_1 == 5 ); 2.7 mm; 2.125 mm))"
equation "parallel_distance_1 = if(( cut_1 == 1 ) or ( cut_1 == 2 ) or ( cut_1 == 3 ) or ( cut_1 == 4 ) or ( cut_1 == 5 ); 4.25 mm; 3.96625 mm)"
equation "pos_2 = round($2)"
equation "cut_2 = if(pos_2 == 1; 1; if(pos_2 == 2; 2; if(pos_2 == 3; 3; if(pos_2 == 4; 4; if(pos_2 == 5; 5; 6)))))"
equation "right_angle_2 = if(cut_2 == 1; 50 deg; if(cut_2 == 2; 65 deg; if(cut_2 == 3; 35 deg; if(cut_2 == 4; 50 deg; if(cut_2 == 5; 65 deg; 65 deg)))))"
equation "left_angle_2 = if(cut_2 == 1; 65 deg; if(cut_2 == 2; 50 deg; if(cut_2 == 3; 65 deg; if(cut_2 == 4; 50 deg; if(cut_2 == 5; 35 deg; 65 deg)))))"
equation "end_diameters_2 = if(( cut_2 == 1 ) or ( cut_2 == 2 ); 3.3 mm; if(( cut_2 == 3 ) or ( cut_2 == 4 ) or ( cut_2 == 5 ); 2.7 mm; 2.125 mm))"
equation "parallel_distance_2 = if(( cut_2 == 1 ) or ( cut_2 == 2 ) or ( cut_2 == 3 ) or ( cut_2 == 4 ) or ( cut_2 == 5 ); 4.25 mm; 3.96625 mm)"
equation "pos_3 = round($3)"
equation "cut_3 = if(pos_3 == 1; 1; if(pos_3 == 2; 2; if(pos_3 == 3; 3; if(pos_3 == 4; 4; if(pos_3 == 5; 5; 6)))))"
equation "right_angle_3 = if(cut_3 == 1; 50 deg; if(cut_3 == 2; 65 deg; if(cut_3 == 3; 35 deg; if(cut_3 == 4; 50 deg; if(cut_3 == 5; 65 deg; 65 deg)))))"
equation "left_angle_3 = if(cut_3 == 1; 65 deg; if(cut_3 == 2; 50 deg; if(cut_3 == 3; 65 deg; if(cut_3 == 4; 50 deg; if(cut_3 == 5; 35 deg; 65 deg)))))"
equation "end_diameters_3 = if(( cut_3 == 1 ) or ( cut_3 == 2 ); 3.3 mm; if(( cut_3 == 3 ) or ( cut_3 == 4 ) or ( cut_3 == 5 ); 2.7 mm; 2.125 mm))"
equation "parallel_distance_3 = if(( cut_3 == 1 ) or ( cut_3 == 2 ) or ( cut_3 == 3 ) or ( cut_3 == 4 ) or ( cut_3 == 5 ); 4.25 mm; 3.96625 mm)"
equation "pos_4 = round($4)"
equation "cut_4 = if(pos_4 == 1; 1; if(pos_4 == 2; 2; if(pos_4 == 3; 3; if(pos_4 == 4; 4; if(pos_4 == 5; 5; 6)))))"
equation "right_angle_4 = if(cut_4 == 1; 50 deg; if(cut_4 == 2; 65 deg; if(cut_4 == 3; 35 deg; if(cut_4 == 4; 50 deg; if(cut_4 == 5; 65 deg; 65 deg)))))"
equation "left_angle_4 = if(cut_4 == 1; 65 deg; if(cut_4 == 2; 50 deg; if(cut_4 == 3; 65 deg; if(cut_4 == 4; 50 deg; if(cut_4 == 5; 35 deg; 65 deg)))))"
equation "end_diameters_4 = if(( cut_4 == 1 ) or ( cut_4 == 2 ); 3.3 mm; if(( cut_4 == 3 ) or ( cut_4 == 4 ) or ( cut_4 == 5 ); 2.7 mm; 2.125 mm))"
equation "parallel_distance_4 = if(( cut_4 == 1 ) or ( cut_4 == 2 ) or ( cut_4 == 3 ) or ( cut_4 == 4 ) or ( cut_4 == 5 ); 4.25 mm; 3.96625 mm)"
equation "pos_5 = round($5)"
equation "cut_5 = if(pos_5 == 1; 1; if(pos_5 == 2; 2; if(pos_5 == 3; 3; if(pos_5 == 4; 4; if(pos_5 == 5; 5; 6)))))"
equation "right_angle_5 = if(cut_5 == 1; 50 deg; if(cut_5 == 2; 65 deg; if(cut_5 == 3; 35 deg; if(cut_5 == 4; 50 deg; if(cut_5 == 5; 65 deg; 65 deg)))))"
equation "left_angle_5 = if(cut_5 == 1; 65 deg; if(cut_5 == 2; 50 deg; if(cut_5 == 3; 65 deg; if(cut_5 == 4; 50 deg; if(cut_5 == 5; 35 deg; 65 deg)))))"
equation "end_diameters_5 = if(( cut_5 == 1 ) or ( cut_5 == 2 ); 3.3 mm; if(( cut_5 == 3 ) or ( cut_5 == 4 ) or ( cut_5 == 5 ); 2.7 mm; 2.125 mm))"
equation "parallel_distance_5 = if(( cut_5 == 1 ) or ( cut_5 == 2 ) or ( cut_5 == 3 ) or ( cut_5 == 4 ) or ( cut_5 == 5 ); 4.25 mm; 3.96625 mm)"
equation "pos_6 = round($6)"
equation "cut_6 = if(pos_6 == 1; 1; if(pos_6 == 2; 2; if(pos_6 == 3; 3; if(pos_6 == 4; 4; if(pos_6 == 5; 5; 6)))))"
equation "right_angle_6 = if(cut_6 == 1; 50 deg; if(cut_6 == 2; 65 deg; if(cut_6 == 3; 35 deg; if(cut_6 == 4; 50 deg; if(cut_6 == 5; 65 deg; 65 deg)))))"
equation "left_angle_6 = if(cut_6 == 1; 65 deg; if(cut_6 == 2; 50 deg; if(cut_6 == 3; 65 deg; if(cut_6 == 4; 50 deg; if(cut_6 == 5; 35 deg; 65 deg)))))"
equation "end_diameters_6 = if(( cut_6 == 1 ) or ( cut_6 == 2 ); 3.3 mm; if(( cut_6 == 3 ) or ( cut_6 == 4 ) or ( cut_6 == 5 ); 2.7 mm; 2.125 mm))"
equation "parallel_distance_6 = if(( cut_6 == 1 ) or ( cut_6 == 2 ) or ( cut_6 == 3 ) or ( cut_6 == 4 ) or ( cut_6 == 5 ); 4.25 mm; 3.96625 mm)"
equation "pos_7 = round($7)"
equation "cut_7 = if(pos_7 == 1; 1; if(pos_7 == 2; 2; if(pos_7 == 3; 3; if(pos_7 == 4; 4; if(pos_7 == 5; 5; 6)))))"
equation "right_angle_7 = if(cut_7 == 1; 50 deg; if(cut_7 == 2; 65 deg; if(cut_7 == 3; 35 deg; if(cut_7 == 4; 50 deg; if(cut_7 == 5; 65 deg; 65 deg)))))"
equation "left_angle_7 = if(cut_7 == 1; 65 deg; if(cut_7 == 2; 50 deg; if(cut_7 == 3; 65 deg; if(cut_7 == 4; 50 deg; if(cut_7 == 5; 35 deg; 65 deg)))))"
equation "end_diameters_7 = if(( cut_7 == 1 ) or ( cut_7 == 2 ); 3.3 mm; if(( cut_7 == 3 ) or ( cut_7 == 4 ) or ( cut_7 == 5 ); 2.7 mm; 2.125 mm))"
equation "parallel_distance_7 = if(( cut_7 == 1 ) or ( cut_7 == 2 ) or ( cut_7 == 3 ) or ( cut_7 == 4 ) or ( cut_7 == 5 ); 4.25 mm; 3.96625 mm)"
equation "pos_8 = round($8)"
equation "cut_8 = if(pos_8 == 1; 1; if(pos_8 == 2; 2; if(pos_8 == 3; 3; if(pos_8 == 4; 4; if(pos_8 == 5; 5; 6)))))"
equation "right_angle_8 = if(cut_8 == 1; 50 deg; if(cut_8 == 2; 65 deg; if(cut_8 == 3; 35 deg; if(cut_8 == 4; 50 deg; if(cut_8 == 5; 65 deg; 65 deg)))))"
equation "left_angle_8 = if(cut_8 == 1; 65 deg; if(cut_8 == 2; 50 deg; if(cut_8 == 3; 65 deg; if(cut_8 == 4; 50 deg; if(cut_8 == 5; 35 deg; 65 deg)))))"
equation "end_diameters_8 = if(( cut_8 == 1 ) or ( cut_8 == 2 ); 3.3 mm; if(( cut_8 == 3 ) or ( cut_8 == 4 ) or ( cut_8 == 5 ); 2.7 mm; 2.125 mm))"
equation "parallel_distance_8 = if(( cut_8 == 1 ) or ( cut_8 == 2 ) or ( cut_8 == 3 ) or ( cut_8 == 4 ) or ( cut_8 == 5 ); 4.25 mm; 3.96625 mm)"
equation "pos_9 = round($9)"
equation "cut_9 = if(pos_9 == 1; 1; if(pos_9 == 2; 2; if(pos_9 == 3; 3; if(pos_9 == 4; 4; if(pos_9 == 5; 5; 6)))))"
equation "right_angle_9 = if(cut_9 == 1; 50 deg; if(cut_9 == 2; 65 deg; if(cut_9 == 3; 35 deg; if(cut_9 == 4; 50 deg; if(cut_9 == 5; 65 deg; 65 deg)))))"
equation "left_angle_9 = if(cut_9 == 1; 65 deg; if(cut_9 == 2; 50 deg; if(cut_9 == 3; 65 deg; if(cut_9 == 4; 50 deg; if(cut_9 == 5; 35 deg; 65 deg)))))"
equation "end_diameters_9 = if(( cut_9 == 1 ) or ( cut_9 == 2 ); 3.3 mm; if(( cut_9 == 3 ) or ( cut_9 == 4 ) or ( cut_9 == 5 ); 2.7 mm; 2.125 mm))"
equation "parallel_distance_9 = if(( cut_9 == 1 ) or ( cut_9 == 2 ) or ( cut_9 == 3 ) or ( cut_9 == 4 ) or ( cut_9 == 5 ); 4.25 mm; 3.96625 mm)"
equation "d65 = d64"
equation "d67 = d66"
equation "d69 = d68"
equation "d70 = d68"
equation "d71 = d68"
equation "d73 = d72"
equation "d74 = d72"
equation "d75 = d72"
equation "d81 = -( 2.57 mm + 35 mm + 2 mm + 3 mm )"
equation "d83 = d64"
equation "d87 = d86"
equation "d90 = d89"
equation "d93 = -( -17.625 mm - 6 mm )"
equation "d101 = d99 / 2"
equation "d104 = d99 / 2"
equation "d110 = d109"
equation "d117 = d64"
equation "d118 = d64"
equation "d119 = d66"
equation "d120 = d66"
equation "d122 = d64 * 2"
equation "d123 = right_angle_1"
equation "d124 = left_angle_1"
equation "d125 = end_diameters_1"
equation "d126 = parallel_distance_1"
equation "d127 = parallel_distance_1"
equation "d128 = d64 * 2.5"
equation "d129 = right_angle_2"
equation "d130 = left_angle_2"
equation "d131 = parallel_distance_2"
equation "d132 = parallel_distance_2"
equation "d133 = end_diameters_2"
equation "d134 = d128"
equation "d135 = right_angle_3"
equation "d136 = left_angle_3"
equation "d137 = parallel_distance_3"
equation "d138 = parallel_distance_3"
equation "d139 = end_diameters_3"
equation "d140 = d128"
equation "d141 = right_angle_4"
equation "d142 = left_angle_4"
equation "d143 = parallel_distance_4"
equation "d144 = parallel_distance_4"
equation "d145 = end_diameters_4"
equation "d146 = d128"
equation "d147 = right_angle_5"
equation "d148 = left_angle_5"
equation "d149 = parallel_distance_5"
equation "d150 = parallel_distance_5"
equation "d151 = end_diameters_5"
equation "d152 = d128"
equation "d156 = d155"
equation "d158 = d128"
equation "d159 = right_angle_6"
equation "d160 = left_angle_6"
equation "d161 = parallel_distance_6"
equation "d162 = parallel_distance_6"
equation "d163 = end_diameters_6"
equation "d164 = d128"
equation "d165 = right_angle_7"
equation "d166 = left_angle_7"
equation "d167 = parallel_distance_7"
equation "d168 = parallel_distance_7"
equation "d169 = end_diameters_7"
equation "d170 = d128"
equation "d171 = right_angle_8"
equation "d172 = left_angle_8"
equation "d173 = parallel_distance_8"
equation "d174 = parallel_distance_8"
equation "d175 = end_diameters_8"
equation "d176 = d128"
equation "d177 = right_angle_9"
equation "d178 = left_angle_9"
equation "d179 = parallel_distance_9"
equation "d180 = parallel_distance_9"
equation "d181 = end_diameters_9"
equation "d182 = d128"
equation "d188 = -2.07 mm - ( 1.5 * 1 mm )"
equation "d191 = -2.07 mm - ( 1.5 * 2 mm )"
equation "d194 = -2.07 mm - ( 1.5 * 3 mm )"
equation "d197 = -2.07 mm - ( 1.5 * 4 mm )"
equation "d200 = -2.07 mm - ( 1.5 * 5 mm )"
equation "d203 = -2.07 mm - ( 1.5 * 6 mm )"
equation "d206 = -2.07 mm - ( 1.5 * 8 mm )"
equation "d209 = -2.07 mm - ( 1.5 * 9 mm )"
equation "d212 = -2.07 mm - ( 1.5 * 10 mm )"
